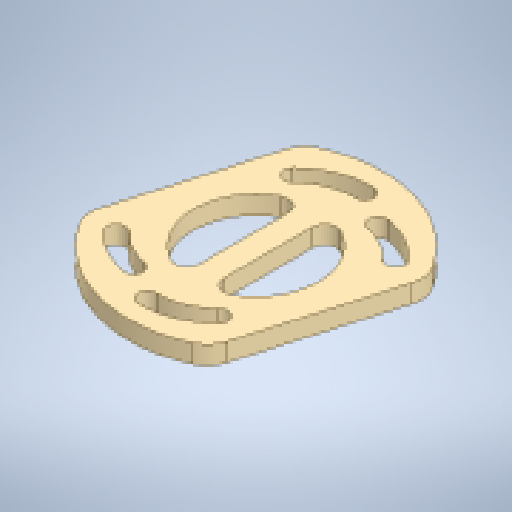
# Autodesk Inventor part: krepezh
Saved by Autodesk Inventor 2024 (Build 280153000, 153)
## iProperties
Created: 2026-02-21
Part Number: krepezh
Material: Типовые
Document SubType Name: Modeling
Designer: akap
Density: 1 g/cm^3
Appearance: Пшеничный
Author: akap
Autodesk Inventor part; units mm, degrees
ref_plane "YZ Plane" through (0, 0, 0) normal (1, 0, 0) x (0, 1, 0)
ref_plane "XZ Plane" through (0, 0, 0) normal (0, 1, 0) x (-1, 0, 0)
ref_plane "XY Plane" through (0, 0, 0) normal (0, 0, 1) x (1, 0, 0)
sketch "Эскиз1" plane through (0, 0, 0) normal (0, 1, 0) x (-1, 0, 0)
  line L0 (-7, 13.1) -> (7, 13.1) construction
  line L1 (7, 13.1) -> (7, -13.1) construction
  line L2 (7, -13.1) -> (-7, -13.1) construction
  line L3 (-7, -13.1) -> (-7, 13.1) construction
  line L4 (-7, 13.1) -> (7, -13.1) construction
  line L5 (7, 13.1) -> (-7, -13.1) construction
  line L6 (-1.437822, -16.490381) -> (13.562178, 9.490381) construction
  line L7 (13.562178, 9.490381) -> (1.437822, 16.490381) construction
  line L8 (1.437822, 16.490381) -> (-13.562178, -9.490381) construction
  line L9 (-13.562178, -9.490381) -> (-1.437822, -16.490381) construction
  line L10 (-1.437822, -16.490381) -> (1.437822, 16.490381) construction
  line L11 (13.562178, 9.490381) -> (-13.562178, -9.490381) construction
  circle A0 centre (13.562178, 9.490381) radius 1.5
  circle A1 centre (1.437822, 16.490381) radius 1.5
  circle A2 centre (7, 13.1) radius 1.5
  circle A3 centre (-7, 13.1) radius 1.5
  circle A4 centre (-7, -13.1) radius 1.5
  circle A5 centre (7, -13.1) radius 1.5
  circle A6 centre (-1.437822, -16.490381) radius 1.5
  circle A7 centre (-13.562178, -9.490381) radius 1.5
  circle A8 centre (0, 0) radius 13.352946
  circle A9 centre (0, 0) radius 15.052945
  circle A10 centre (0, 0) radius 18.052945
  circle A11 centre (0, 0) radius 16.352946
  circle A12 centre (0, 0) radius 21.052945
  circle A13 centre (0, 0) radius 10.352946
  line L12 (-2, 10.352946) -> (2, 10.352946) construction
  line L13 (2, 10.352946) -> (2, -10.352946)
  line L14 (2, -10.352946) -> (-2, -10.352946) construction
  line L15 (-2, -10.352946) -> (-2, 10.352946)
  line L16 (-2, 10.352946) -> (2, -10.352946) construction
  line L17 (2, 10.352946) -> (-2, -10.352946) construction
  circle A14 centre (1.157182, 4.993806) radius 10
  circle A15 centre (1.157182, 4.993806) radius 13
  circle A16 centre (5.040606, 1.768152) radius 10
  circle A17 centre (5.040606, 1.768152) radius 13
  circle A18 centre (-1.157182, -4.993806) radius 10
  circle A19 centre (-1.157182, -4.993806) radius 13
  circle A20 centre (-5.040606, -1.768152) radius 10
  circle A21 centre (-5.040606, -1.768152) radius 13
  point P0 (6.29307, 11.77703)
  point P1 (1.307529, 14.996051)
  point P2 (-1.307529, -14.996051)
  point P3 (-6.29307, -11.77703)
  point P4 (-7.70693, -14.42297)
  point P5 (-6.29307, 11.77703)
  point P6 (-7.70693, 14.42297)
  point P7 (14.79116, 10.350383)
  point P8 (12.333196, 8.630379)
  point P9 (6.29307, -11.77703)
  point P10 (7.70693, -14.42297)
  point P11 (-14.79116, -10.350383)
  point P12 (-12.333196, -8.630379)
  point P13 (-2, 10.157927)
  point P14 (-2, -10.157927)
  point P15 (2, -10.157927)
  point P16 (2, 10.157927)
  point P17 (8.377519, -12.506332)
  point P18 (-14.189914, -8.128049)
  point P19 (14.189914, 8.128049)
  point P20 (-8.377519, 12.506332)
  point P21 (7.255573, 14.578067)
  point P22 (14.673687, 10.497628)
  point P23 (12.387672, 8.552003)
  point P24 (6.744427, 11.621933)
  point P25 (6.398093, -8.139281)
  point P26 (6.282627, -8.154417)
  point P27 (6.207779, -8.285346)
  point P28 (8.06398, -14.15733)
  point P29 (-1.474427, -17.989934)
  point P30 (-1.354811, -14.991853)
  point P31 (5.93602, -12.04267)
  point P32 (-7.255573, -14.578067)
  point P33 (-14.673687, -10.497628)
  point P34 (-12.387672, -8.552003)
  point P35 (-6.744427, -11.621933)
  point P36 (1.354811, 14.991853)
  point P37 (-5.93602, 12.04267)
  point P38 (-8.06398, 14.15733)
  point P39 (1.474427, 17.989934)
  dimension "d6" = 3
  dimension "d7" = 3
  dimension "d11" = 3
  dimension "d0" = 14
  dimension "d1" = 26.2
  dimension "d2" = 30
  dimension "d3" = 14
  dimension "d5" = 3
  dimension "d8" = 3
  dimension "d9" = 3
  dimension "d10" = 3
  dimension "d12" = 3
  dimension "d15" = 3
  dimension "d16" = 3
  dimension "d19" = 3
  dimension "d22" = 3
  dimension "d23" = 4
  dimension "d26" = 30
  dimension "d28" = 20
  dimension "d29" = 3
  dimension "d30" = 20
  dimension "d31" = 3
  dimension "d32" = 20
  dimension "d33" = 3
  dimension "d34" = 20
  dimension "d35" = 3
  constraints: 36 end point, 18 centre point, 10 coincident, 6 midpoint, 6 parallel, 6 point on circle, 6 tangent, 3 perpendicular, 2 horizontal, 17 other
  measures "d0" distance of L1.end L2.end
  measures "d1" distance of L0.end L1.end
  measures "d2" distance of L6.start L6.end
  measures "d3" distance of L7.end L6.end
  measures "d5" diameter of A0
  measures "d8" diameter of A3
  measures "d9" diameter of A4
  measures "d10" diameter of A5
  measures "d12" diameter of A7
  measures "d15" radial gap between concentric circles of A9 A10
  measures "d19" radial gap between concentric circles of A10 A12
  measures "d22" radial gap between concentric circles of A8 A13
  measures "d23" distance of L13.end L14.end
  measures "d26" angle of L3 L8
  measures "d28" diameter of A14
  measures "d29" radial gap between concentric circles of A14 A15
  measures "d30" diameter of A16
  measures "d31" radial gap between concentric circles of A16 A17
  measures "d32" diameter of A18
  measures "d33" radial gap between concentric circles of A18 A19
  measures "d34" diameter of A20
  measures "d35" radial gap between concentric circles of A20 A21
extrude "Выдавливание1" add sketch "Эскиз1" along normal blind 3 contours A0 A10 A17 A11 | A10 A17 | A0 A17 A10 | A11 A17 A9 A16 A15 A0 | A17 A15 A10 | A10 A6 A19 A11 A17 | A15 A16 A0 | A17 A11 A1 A10 A15 | A11 A19 A9 A17 | A10 A1 A15 | A16 A9 A0 | A16 A15 A9 | A16 A9 A15 | A17 A14 A1 A11 | A19 A10 A6 | A17 A19 A8 A16 A9 | A9 A19 A17 | A1 A15 A11 A21 A10 | A9 A15 A8 A14 A16 | A9 A16 A8 A15 | A2 A9 A14 A17 | A10 A19 A21 A11 A6 | A10 A21 A19 | A5 A9 A19 | A9 A5 A8 A17 A19 | A17 A8 A19 | A21 A11 A7 A10 | A10 A21 | A14 A8 A16 | A14 A17 A9 A1 | A2 A14 A9 | A14 A9 A17 | A11 A21 A18 A6 | A10 A7 A21 | A5 A18 A8 | A17 A18 A16 A19 A8 | A8 A18 A17 | A19 A16 A8 | A15 A9 A21 A11 | A21 A9 A20 A19 A7 A11 | A8 A16 A13 A21 A17 | A14 A19 A13 A16 A8 | A8 A15 A19 A14 | A16 A8 A2 | A16 A19 A15 A8 | A9 A17 A8 A14 | A2 A8 A17 A9 A14 | A18 A21 A9 A6 | A18 A9 A21 A8 | A18 A8 A21 A17 | A17 A21 A13 A16 A18 | A16 A18 A15 A19 | A3 A9 A15 | A21 A15 A8 A20 A9 | A9 A15 A21 | A15 A18 A13 A14 A19 | A8 A14 A21 | A8 A21 A15 A9 A3 | A14 A8 A3 | A17 A21 A14 A8 | A21 A4 A9 A18 | A18 A9 A21 | A8 A21 A9 A18 A4 | A21 A8 A20 A13 A17 | A17 A13 A21 | A16 A13 A15 A18 | A19 A20 A7 | A20 A8 A19 A9 | A9 A19 A20 | A21 A8 A15 | A16 A21 A13 | A13 L13 A21 A16 | A14 A13 A19 | A15 A13 A18 | A21 A13 A17 | A17 A13 A20 A14 A21 | A9 A4 A18 | A17 A20 L13 A13 | A13 A20 A17 | A20 A9 A7 | A20 A19 A9 | A19 A8 A18 A20 A9 | A20 A15 A19 A8 | A8 A15 A20 | A8 A21 A14 A20 A15 | A21 A16 L15 A13 | A21 L13 A19 L15 A16 | A4 A20 A8 | A20 A8 A18 A15 A13 | A13 L15 A17 A20 | A17 L15 A15 L13 A20 | A19 A15 A18 A8 | A20 A14 A19 A15 | A20 A13 A19 A14 | A20 A18 A8 | A19 A14 A13 A18 A15 | L13 A20 L15 A19 | A19 A13 A14 | A15 A18 A13 | A15 L15 A16 L13 | L13 A18 L15 A20 | A16 L15 A14 L13 | L13 A14 L15 A18 | A12 picked at (5.651458, 13.934035) picked at (-0.217232, 10.33749) picked at (-5.651458, -13.934035) picked at (0.217232, -10.33749)
fillet "Сопряжение1" radius 2 4 edges at (-2, 1.5, -10.1579) (-2, 1.5, 10.1579) (2, 1.5, 10.1579) (2, 1.5, -10.1579)
sketch "Эскиз2" plane through (0, 3, 0) normal (0, 1, 0) x (1, 0, 0)
  line L0 (-18.777493, -9.520098) -> (-10.754619, 18.098748)
  circle A0 centre (0, 0) radius 21.052945
  line L1 (10.754619, -18.098748) -> (18.777493, 9.520098)
  line L2 (0, 0) -> (0, 4.178964)
  line L3 (-18.777493, -9.520098) -> (10.754619, -18.098748) construction
  arc A1 (-12.333196, -8.630379) -> (-14.673687, -10.497628) centre (-13.562178, -9.490381) ccw
  arc A2 (-8.06398, 14.15733) -> (-5.93602, 12.04267) centre (-7, 13.1) ccw
  dimension "d38" = 5
  dimension "d40" = 5
  constraints: 8 end point, 4 point on circle, 1 parallel, 1 perpendicular, 1 vertical
  measures "d38" distance from line of L0 A1.centre
  measures "d40" distance from line of L0 A2.centre
extrude "Выдавливание2" cut sketch "Эскиз2" against normal blind 3 contours A0 L0 | L1 A0
fillet "Сопряжение2" radius 5 4 edges at (-18.7775, 1.5, 9.5201) (-10.7546, 1.5, -18.0987) (18.7775, 1.5, -9.5201) (10.7546, 1.5, 18.0987)
